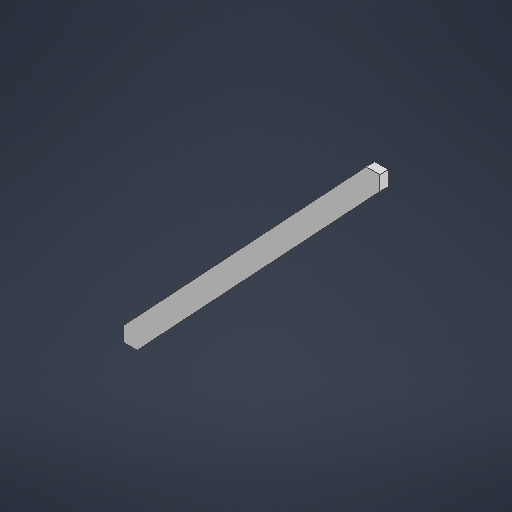
# Autodesk Inventor part: S_2x4x64.444
Saved by Autodesk Inventor 2026 (Build 300175000, 175)
## iProperties
Created: 2025-09-09
Part Number: S_2x4x64.444
Material: Generic
Document SubType Name: Modeling
Designer: trott
Density: 1 g/cm^3
Appearance: Default
Author: trott
Autodesk Inventor part; units mm, degrees
ref_plane "YZ Plane" through (0, 0, 0) normal (1, 0, 0) x (0, 1, 0)
ref_plane "XZ Plane" through (0, 0, 0) normal (0, 1, 0) x (-1, 0, 0)
ref_plane "XY Plane" through (0, 0, 0) normal (0, 0, 1) x (1, 0, 0)
sketch "Sketch1" plane through (0, 0, 0) normal (0, 0, 1) x (1, 0, 0)
  line L0 (-571.5, -609.6) -> (571.5, -609.6)
  line L1 (571.5, -609.6) -> (571.5, 609.6)
  line L2 (571.5, 609.6) -> (-571.5, 609.6)
  line L3 (-571.5, 609.6) -> (-571.5, -609.6)
  line L4 (-571.5, -609.6) -> (571.5, 609.6) construction
  line L5 (571.5, -609.6) -> (-571.5, 609.6) construction
  line L6 (571.5, 609.6) -> (-571.5, -609.6)
  line L7 (-539.0721, -640.0012) -> (-603.9279, -579.1988)
  line L8 (603.9279, 579.1988) -> (539.0721, 640.0012)
  line L9 (539.0721, 640.0012) -> (-603.9279, -579.1988)
  line L10 (603.9279, 579.1988) -> (-539.0721, -640.0012)
  point P0 (0, 0)
  point P1 (510.571, 609.6)
  point P2 (-571.5, -544.609)
  point P3 (-510.571, -609.6)
  point P4 (571.5, 544.609)
  dimension "d0" = 1143
  dimension "d1" = 1219.2
  dimension "d2" = 88.9
  dimension "d3" = 88.9
  constraints: 22 end point, 4 midpoint, 3 equal length, 3 perpendicular, 1 horizontal
  measures "d0" distance of L2.end L1.end
  measures "d1" distance of L0.end L1.end
  measures "d2" distance of L7.start L7.end
  measures "d3" distance of L8.start L8.end
extrude "Extrusion1" add sketch "Sketch1" along normal blind 38.1 contours L6 L1 L10 L0 | L3 L9 L2 L6
body "Solid1"
